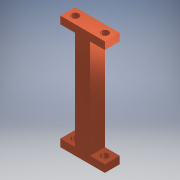
# Autodesk Inventor part: shaft
Saved by Autodesk Inventor 2017 (Build 210142000, 142)
## iProperties
Created: 2019-12-06
Part Number: shaft
Material: Generic
Document SubType Name: Modeling
Designer: User
Density: 1 g/cm^3
Appearance: Default
Mass: 2.00318 g
Surface Area: 16.6455 cm^2
Volume: 2.00318 cm^3
Author: User
Autodesk Inventor part; units mm, degrees
ref_plane "YZ Plane" through (0, 0, 0) normal (1, 0, 0) x (0, 1, 0)
ref_plane "XZ Plane" through (0, 0, 0) normal (0, 1, 0) x (-1, 0, 0)
ref_plane "XY Plane" through (0, 0, 0) normal (0, 0, 1) x (1, 0, 0)
sketch "Sketch1" plane through (0, 0, 0) normal (0, 0, 1) x (1, 0, 0)
  line L0 (-9, -3) -> (9, -3)
  line L1 (9, -3) -> (9, 3)
  line L2 (9, 3) -> (-9, 3)
  line L3 (-9, 3) -> (-9, -3)
  line L4 (-9, -3) -> (9, 3) construction
  line L5 (9, -3) -> (-9, 3) construction
  point P0 (0, 0)
  dimension "d0" = 18
  dimension "d1" = 6
  constraints: 12 end point, 2 midpoint, 2 parallel, 1 horizontal, 1 perpendicular
  measures "d0" distance of L2.end L1.end
  measures "d1" distance of L1.end L0.end
extrude "Extrusion1" add sketch "Sketch1" along normal blind 3
sketch "Sketch2" plane through (0, 0, 3) normal (0, 0, 1) x (1, 0, 0)
  line L0 (-3, 3) -> (3, 3)
  line L1 (3, 3) -> (3, -3)
  line L2 (3, -3) -> (-3, -3)
  line L3 (-3, -3) -> (-3, 3)
  line L4 (-3, 3) -> (3, -3) construction
  line L5 (3, 3) -> (-3, -3) construction
  point P0 (0, 0)
  dimension "d4" = 6
  dimension "d5" = 6
  constraints: 12 end point, 2 midpoint, 2 parallel, 1 horizontal, 1 perpendicular
  measures "d4" distance of L1.end L2.end
  measures "d5" distance of L0.end L1.end
extrude "Extrusion2" add sketch "Sketch2" along normal blind 40
sketch "Sketch3" plane through (0, 0, 43) normal (0, 0, 1) x (1, 0, 0)
  line L0 (9, 3) -> (-9, 3) projected
  line L1 (9, -3) -> (-9, -3)
  line L2 (-9, -3) -> (-9, 3)
  line L3 (-9, 3) -> (9, 3)
  line L4 (9, 3) -> (9, -3)
  line L5 (9, -3) -> (-9, 3) construction
  line L6 (-9, -3) -> (9, 3) construction
  point P0 (0, 0)
  constraints: 12 end point, 2 midpoint, 2 parallel, 1 horizontal, 1 perpendicular
extrude "Extrusion3" add sketch "Sketch3" along normal blind 3
sketch "Sketch4" plane through (0, 0, 46) normal (0, 0, 1) x (1, 0, 0)
  circle A0 centre (6, 0) radius 1.5
  circle A1 centre (-6, 0) radius 1.5
  point P0 (0, 0)
  dimension "d10" = 3
  dimension "d11" = 3
  constraints: 2 centre point
  measures "d10" diameter of A0
  measures "d11" diameter of A1
extrude "Extrusion4" cut sketch "Sketch4" against normal up to surface (46 mm away)
body "Solid1"
